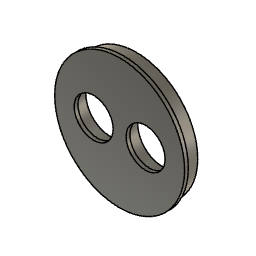
deksel airgap v2 (Autodesk Fusion 360 design; units mm, degrees)
Autodesk Fusion 360 part; units mm, degrees
sketch "Sketch1" plane through (0, 0, 0) normal (0, 1, 0) x (1, 0, 0)
  circle A0 centre (0, 0) radius 33.075
  circle A1 centre (0, 0) radius 35
  dimension "d1" = 66.15
  dimension "d2" = 70
  constraint coincident A0.centre A1.centre
  measures "d1" diameter of A0
  measures "d2" diameter of A1
extrude "Extrude1" add sketch "Sketch1" along normal blind 7 contours A0
extrude "Extrude2" add sketch "Sketch1" against normal blind 2 contours A0 | A1
sketch "Sketch4" plane through (0, -2, 0) normal (0, -1, 0) x (1, 0, 0)
  circle A0 centre (0, 0) radius 35
  circle A1 centre (14, 0) radius 10.5
  circle A2 centre (0, 0) radius 33.075
  dimension "d33" = 21
  dimension "d39" = 14
  measures "d33" diameter of A1
  measures "d39" distance of A1.centre A0.centre
extrude "Extrude8" cut sketch "Sketch4" against normal up to surface (9 mm away) contours A1
sketch "Sketch5" plane through (0, 7, 0) normal (0, 1, 0) x (-1, 0, 0)
  circle A0 centre (-14, 0) radius 10.5
  circle A1 centre (0, 0) radius 33.075
  circle A2 centre (-14, 0) radius 13.25
  dimension "d36" = 26.5
  constraint concentric A0 A2
  measures "d36" diameter of A2
extrude "Extrude9" cut sketch "Sketch5" against normal blind 7 contours A2
mirror "Mirror3" about plane through (0, 0, 0) normal (1, 0, 0) of "Extrude8", "Extrude9"
